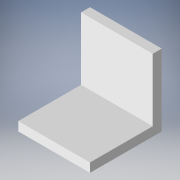
# Autodesk Inventor part: 15102898-16-P-0313
Saved by Autodesk Inventor 2017 (Build 210142000, 142)
## iProperties
Created: 2016-11-05
Part Number: 15102898-16-P-0313
Material: Generic
Document SubType Name: Modeling
Designer: gus
Density: 1 g/cm^3
Appearance: Default
Author: gus
Autodesk Inventor part; units mm, degrees
ref_plane "YZ Plane" through (0, 0, 0) normal (1, 0, 0) x (0, 1, 0)
ref_plane "XZ Plane" through (0, 0, 0) normal (0, 1, 0) x (-1, 0, 0)
ref_plane "XY Plane" through (0, 0, 0) normal (0, 0, 1) x (1, 0, 0)
sketch "Sketch1" plane through (0, 0, 0) normal (1, 0, 0) x (0, 1, 0)
  line L0 (0, 0) -> (25.4, 0)
  line L1 (25.4, 0) -> (25.4, 3.175)
  line L2 (25.4, 3.175) -> (3.175, 3.175)
  line L3 (3.175, 3.175) -> (3.175, 25.4)
  line L4 (3.175, 25.4) -> (0, 25.4)
  line L5 (0, 25.4) -> (0, 0)
  dimension "d0" = 25.4
  dimension "d1" = 25.4
  dimension "d2" = 3.175
  dimension "d3" = 3.175
  constraints: 12 end point, 5 perpendicular, 1 horizontal
  measures "d0" distance of L4.end L0.start
  measures "d1" distance of L0.start L0.end
  measures "d2" distance of L0.end L1.end
  measures "d3" distance of L3.end L4.end
extrude "Extrusion1" add sketch "Sketch1" along normal blind 25.4
sketch "Sketch2" plane through (0, 3.175, 3.175) normal (0, 0, 1) x (1, 0, 0)
  line L0 (25.4, -3.175) -> (25.4, 22.225) projected
  line L1 (0, 22.225) -> (25.4, 22.225) projected
  point P0 (0, -3.175)
  point P1 (12.7, 15.875)
  dimension "d6" = 12.7
  dimension "d7" = 6.35
  measures "d6" distance from line of L0 point (12.7, 15.875)
  measures "d7" distance from line of L1 point (12.7, 15.875)
hole "Hole1" at (12.7, 19.05, 3.175) direction (0, 0, -1) diameter 6.7469 end through all
sketch "Sketch3" plane through (0, 3.175, 25.4) normal (0, 1, 0) x (1, 0, 0)
  line L0 (0, 25.4) -> (25.4, 25.4) projected
  line L1 (25.4, 22.225) -> (25.4, 0) projected
  point P0 (12.7, 12.7)
  dimension "d15" = 12.7
  dimension "d16" = 12.7
  measures "d15" distance from line of L0 point (12.7, 12.7)
  measures "d16" distance from line of L1 point (12.7, 12.7)
hole "Hole2" at (12.7, 3.175, 12.7) direction (0, -1, 0) diameter 12.7 end through all
body "Solid1"
